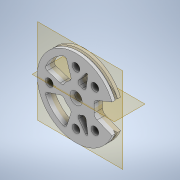
# Autodesk Inventor part: tendon_wh_2
Saved by Autodesk Inventor 2020 (Build 240168000, 168)
## iProperties
Created: 2020-12-06
Part Number: tendon_wh_2
Material: Generic
Document SubType Name: Modeling
Designer: Shuang Peng
Density: 1 g/cm^3
Appearance: Default
Mass: 3.1357 g
Surface Area: 22.5566 cm^2
Volume: 3.1357 cm^3
Author: Shuang Peng
Autodesk Inventor part; units mm, degrees
ref_plane "YZ Plane" through (0, 0, 0) normal (1, 0, 0) x (0, 1, 0)
ref_plane "XZ Plane" through (0, 0, 0) normal (0, 1, 0) x (-1, 0, 0)
ref_plane "XY Plane" through (0, 0, 0) normal (0, 0, 1) x (1, 0, 0)
sketch "Sketch1" plane through (0, 0, 0) normal (0, 0, 1) x (1, 0, 0)
  circle A0 centre (13.788582, -13.788582) radius 1.5
  circle A1 centre (0, 0) radius 3
  circle A2 centre (13.788582, -13.788582) radius 16
  point P0 (0, 0)
  dimension "d0" = 32
  constraints: 1 centre point, 1 coincident
  measures "d0" diameter of A2
extrude "Extrusion1" add sketch "Sketch1" along normal blind 3.5 contours A0 | A2
sketch "Sketch2" plane through (13.788582, -13.788582, 0) normal (0, 0, -1) x (-1, 0, 0)
  circle A0 centre (0, 0) radius 3.075
  line L0 (11.788582, 25.288582) -> (11.788582, 22.395184)
  line L1 (11.788582, 22.395184) -> (5.181981, 15.788582)
  line L2 (5.181981, 15.788582) -> (2.288582, 15.788582)
  arc A1 (2.288582, 15.788582) -> (0.510961, 14.705131) centre (2.288582, 13.788582) ccw
  line L3 (0.510961, 14.705131) -> (-7.071068, 0)
  line L4 (-7.071068, 0) -> (0, -7.071068)
  line L5 (0, -7.071068) -> (14.705131, 0.510961)
  arc A2 (14.705131, 0.510961) -> (15.788582, 2.288582) centre (13.788582, 2.288582) ccw
  line L6 (15.788582, 2.288582) -> (15.788582, 5.181981)
  line L7 (15.788582, 5.181981) -> (22.395184, 11.788582)
  line L8 (22.395184, 11.788582) -> (25.288582, 11.788582)
  arc A3 (25.288582, 11.788582) -> (25.288582, 15.788582) centre (25.288582, 13.788582) ccw
  line L9 (25.288582, 15.788582) -> (22.395184, 15.788582)
  line L10 (22.395184, 15.788582) -> (15.788582, 22.395184)
  line L11 (15.788582, 22.395184) -> (15.788582, 25.288582)
  arc A4 (15.788582, 25.288582) -> (11.788582, 25.288582) centre (13.788582, 25.288582) ccw
  circle A5 centre (13.788582, 25.288582) radius 1
  circle A6 centre (25.288582, 13.788582) radius 1
  circle A7 centre (13.788582, 13.788582) radius 5.15
  circle A8 centre (13.788582, 2.288582) radius 1
  circle A9 centre (2.288582, 13.788582) radius 1
  circle A10 centre (13.788582, 13.788582) radius 13.55
  circle A11 centre (0, 0) radius 4
  point P0 (13.788582, 13.788582)
  dimension "d3" = 8
  constraints: 1 centre point, 1 coincident
  measures "d3" diameter of A11
ref_plane "Work Plane1" through (5.684582, -20.85965, -8) normal (0, 0, 1) x (1, 0, 0)
extrude "Extrusion2" add sketch "Sketch2" along normal up to surface (8 mm away) contours A0 | A11
sketch "Sketch3" plane through (13.788582, -13.788582, -8) normal (0, 0, -1) x (-1, 0, 0)
  circle A0 centre (0, 0) radius 4 projected
  circle A1 centre (0, 0) radius 1.5
  point P0 (13.788582, 13.788582)
  dimension "d6" = 3
  constraints: 1 centre point, 1 coincident
  measures "d6" diameter of A1
extrude "Extrusion3" cut sketch "Sketch3" against normal blind 20 contours A1
ref_plane "Work Plane2" through (13.788582, -13.788582, 1.75) normal (0, 0, 1) x (1, 0, 0)
sketch "Sketch4" plane through (13.788582, -13.788582, 0) normal (0, 0, -1) x (-1, 0, 0)
  circle A0 centre (0, 0) radius 4 projected
  circle A1 centre (0, 0) radius 16 projected
  line L0 (0, 0) -> (10, 0)
  line L1 (11.5, 1.5) -> (8.5, 1.5)
  line L2 (8.5, 1.5) -> (8.5, -1.5)
  line L3 (8.5, -1.5) -> (11.5, -1.5)
  line L4 (11.5, -1.5) -> (11.5, 1.5)
  line L5 (11.5, 1.5) -> (8.5, -1.5) construction
  line L6 (8.5, 1.5) -> (11.5, -1.5) construction
  point P0 (13.788582, 13.788582)
  dimension "d9" = 10
  dimension "d10" = 3
  dimension "d11" = 3
  constraints: 14 end point, 2 midpoint, 2 parallel, 2 perpendicular, 1 horizontal
  measures "d9" distance of L0.start L0.end
  measures "d10" distance of L1.start L1.end
  measures "d11" distance of L2.end L1.end
extrude "Extrusion4" cut sketch "Sketch4" against normal blind 20 contours L4 L3 L2 L1
ref_plane "Work Plane3" through (2.288582, -13.788582, 0) normal (0, -1, 0) x (1, 0, 0)
sketch "Sketch5" plane through (2.288582, -13.788582, 0) normal (0, -1, 0) x (1, 0, 0)
  line L0 (27.5, 3.5) -> (-4.5, 3.5) projected
  line L1 (27.5, 0) -> (-4.5, 0) projected
  line L2 (-4.5, 0) -> (-4.5, 3.5)
  line L3 (-4.5, 0) -> (-4.5, 3.5) projected
  line L4 (-4.5, 1.75) -> (-4.5, 2.25)
  line L5 (-4.5, 1.75) -> (-4, 1.75)
  line L6 (-4.5, 1.75) -> (-4.5, 1.25)
  line L7 (-4.5, 1.25) -> (-4, 1.75)
  line L8 (-4.5, 2.25) -> (-4, 1.75)
  line L9 (15.5, 0) -> (7.5, 0) projected
  line L10 (7.5, -8) -> (15.5, -8) projected
  line L11 (11.5, 0) -> (11.5, -20)
  point P0 (-2.288582, 0)
  dimension "d15" = 0.5
  dimension "d16" = 0.5
  dimension "d17" = 0.5
  dimension "d18" = 20
  constraints: 14 end point, 2 midpoint, 2 point on line, 1 collinear, 1 horizontal, 1 vertical
  measures "d15" distance of L4.start L4.end
  measures "d16" distance of L4.start L5.end
  measures "d17" distance of L4.start L6.end
  measures "d18" distance of L11.start L11.end
revolve "Revolution1" cut sketch "Sketch5" angle 360 about axis through (13.788582, -13.788582, 0) along (0, 0, -1)
sketch "Sketch6" plane through (13.788582, -13.788582, 3.5) normal (0, 0, 1) x (1, 0, 0)
  line L0 (-11.5, 1.5) -> (-8.5, 1.5)
  line L1 (-8.5, 1.5) -> (-8.5, -1.5)
  line L2 (-8.5, -1.5) -> (-11.5, -1.5)
  line L3 (-11.5, -1.5) -> (-11.5, 1.5)
  circle A0 centre (0, 0) radius 1.5
  circle A1 centre (0, 0) radius 16
  line L4 (0, 0) -> (16, 0)
  line L5 (0, 0) -> (11.313708, -11.313708)
  line L6 (0, 0) -> (11.313708, 11.313708)
  line L7 (0, 0) -> (7.778175, -7.778175)
  circle A2 centre (7.778175, -7.778175) radius 1.6
  line L8 (0, 0) -> (7.778175, 7.778175)
  circle A3 centre (7.778175, 7.778175) radius 1.6
  point P0 (-13.788582, 13.788582)
  dimension "d20" = 45
  dimension "d21" = 45
  dimension "d22" = 11
  dimension "d23" = 3.2
  dimension "d24" = 11
  dimension "d25" = 3.2
  constraints: 10 end point, 3 point on circle, 2 centre point, 2 coincident, 2 point on line, 1 horizontal
  measures "d20" angle of L4 L5
  measures "d21" angle of L4 L6
  measures "d22" distance of L4.start L7.end
  measures "d23" diameter of A2
  measures "d24" distance of L4.start L8.end
  measures "d25" diameter of A3
extrude "Extrusion5" cut sketch "Sketch6" against normal blind 20 contours A3 L6 | L6 A3 | A2 L5 | L5 A2
sketch "Sketch7" plane through (13.788582, -13.788582, 3.5) normal (0, 0, 1) x (1, 0, 0)
  circle A0 centre (7.778175, 7.778175) radius 1.6
  circle A1 centre (7.778175, -7.778175) radius 1.6
  line L0 (-11.5, 1.5) -> (-8.5, 1.5)
  line L1 (-8.5, 1.5) -> (-8.5, -1.5)
  line L2 (-8.5, -1.5) -> (-11.5, -1.5)
  line L3 (-11.5, -1.5) -> (-11.5, 1.5)
  circle A2 centre (0, 0) radius 1.5
  circle A3 centre (0, 0) radius 16
  line L4 (0, 0) -> (16, 0)
  line L5 (0, 0) -> (14.834942, 5.993705)
  line L6 (0, 0) -> (14.834942, -5.993705)
  line L7 (7.417471, -2.996853) -> (7.417471, 2.996853)
  point P0 (-13.788582, 13.788582)
  dimension "d28" = 22
  dimension "d29" = 22
  constraints: 8 end point, 3 point on circle, 2 midpoint, 1 horizontal
  measures "d28" angle of L4 L6
  measures "d29" angle of L4 L5
extrude "Extrusion6" cut sketch "Sketch7" against normal blind 20 contours L7 L5 A3 L4 | L4 A3 L6 L7
fillet "Fillet1" radius 2 2 edges at (21.2061, -16.7854, 1.75) (21.2061, -10.7917, 1.75)
sketch "Sketch8" plane through (28.623524, -19.782288, 3.5) normal (0.3746066, 0.9271839, 0) x (0.9271839, -0.3746066, 0)
  line L0 (-6.650983, 0) -> (-6.650983, 3.5)
  line L1 (0, 0) -> (-6.650983, 0)
  line L2 (0, 1.25) -> (0, 0)
  line L3 (-0.5, 1.75) -> (0, 1.25)
  line L4 (0, 2.25) -> (-0.5, 1.75)
  line L5 (0, 3.5) -> (0, 2.25)
  line L6 (-6.650983, 3.5) -> (0, 3.5)
  line L7 (-0.5, 1.75) -> (-1.2, 1.75)
  line L8 (-31.5, 1.75) -> (-0.5, 1.75)
  line L9 (-1.2, 1.75) -> (0, 1.25)
  line L10 (0, 2.25) -> (-32, 2.25)
  line L11 (-1.2, 1.75) -> (0, 2.25)
  point P0 (-33.949845, 3.5)
  point P1 (-4.850233, 1.75)
  point P2 (-4.490563, 2.25)
  dimension "d33" = 0.7
  constraints: 6 end point, 1 point on line
  measures "d33" distance of L3.start L7.end
extrude "Extrusion7" cut sketch "Sketch8" against normal blind 20 contours L11 L4 L7 | L7 L3 L9
sketch "Sketch9" plane through (28.623524, -7.794877, 0) normal (0.3746066, -0.9271839, 0) x (0.9271839, 0.3746066, 0)
  line L0 (-6.650983, 0) -> (-6.650983, 3.5)
  line L1 (0, 0) -> (-6.650983, 0)
  line L2 (0, 1.25) -> (0, 0)
  line L3 (-0.5, 1.75) -> (0, 1.25)
  line L4 (0, 2.25) -> (-0.5, 1.75)
  line L5 (0, 3.5) -> (0, 2.25)
  line L6 (-6.650983, 3.5) -> (0, 3.5)
  line L7 (-0.5, 1.75) -> (-1.2, 1.75)
  line L8 (-0.5, 1.75) -> (-31.5, 1.75)
  line L9 (-1.2, 1.75) -> (0, 2.25)
  line L10 (-32, 1.25) -> (0, 1.25)
  line L11 (-1.2, 1.75) -> (0, 1.25)
  point P0 (-23.619257, 0)
  point P1 (-8.552973, 1.75)
  point P2 (-4.490563, 1.25)
  dimension "d36" = 0.7
  constraints: 6 end point, 1 point on line
  measures "d36" distance of L3.start L7.end
extrude "Extrusion8" cut sketch "Sketch9" against normal blind 20 contours L11 L7 L3 | L9 L4 L7
sketch "Sketch10" plane through (0, 0, 0) normal (0, 0, -1) x (-1, 0, 0)
  arc A0 (-25.785678, -23.602842) -> (-25.785678, -3.974323) centre (-13.788582, -13.788582) ccw
  line L0 (-13.788582, -13.788582) -> (-13.788582, -2.788582)
  circle A1 centre (-13.788582, -2.788582) radius 1.6
  line L1 (-13.788582, -13.788582) -> (-13.788582, -24.788582)
  circle A2 centre (-13.788582, -24.788582) radius 1.6
  point P0 (0, 0)
  dimension "d41" = 11
  dimension "d42" = 3.2
  dimension "d43" = 11
  dimension "d44" = 3.2
  constraints: 4 end point, 2 centre point, 2 coincident, 2 vertical
  measures "d41" distance of L0.start L0.end
  measures "d42" diameter of A1
  measures "d43" distance of L0.start L1.end
  measures "d44" diameter of A2
extrude "Extrusion9" cut sketch "Sketch10" against normal blind 20
sketch "Sketch11" plane through (0, 0, 3.5) normal (0, 0, 1) x (1, 0, 0)
  circle A0 centre (13.788582, -2.788582) radius 1.6
  circle A1 centre (13.788582, -24.788582) radius 1.6
  line L0 (28.623524, -19.782288) -> (22.45684, -17.290786)
  arc A2 (21.206053, -15.436418) -> (22.45684, -17.290786) centre (23.206053, -15.436418) ccw
  line L1 (21.206053, -15.436418) -> (21.206053, -12.140747)
  arc A3 (22.45684, -10.286379) -> (21.206053, -12.140747) centre (23.206053, -12.140747) ccw
  line L2 (22.45684, -10.286379) -> (28.623524, -7.794877)
  arc A4 (28.623524, -7.794877) -> (28.623524, -19.782288) centre (13.788582, -13.788582) ccw
  circle A5 centre (13.788582, -13.788582) radius 1.5
  line L3 (2.288582, -12.288582) -> (5.288582, -12.288582)
  line L4 (5.288582, -12.288582) -> (5.288582, -15.288582)
  line L5 (5.288582, -15.288582) -> (2.288582, -15.288582)
  line L6 (2.288582, -15.288582) -> (2.288582, -12.288582)
  circle A6 centre (21.566757, -21.566757) radius 1.6
  circle A7 centre (21.566757, -6.010408) radius 1.6
  point P0 (0, 0)
extrude "Extrusion10" add sketch "Sketch11" against normal up to surface (3.5 mm away) contours L3 L4 L5 L6
sketch "Sketch12" plane through (0, 0, 0) normal (0, 0, -1) x (-1, 0, 0)
  circle A0 centre (-13.788582, -2.788582) radius 1.6
  circle A1 centre (-13.788582, -24.788582) radius 1.6
  line L0 (-22.45684, -17.290786) -> (-28.623524, -19.782288)
  arc A2 (-28.623524, -19.782288) -> (-28.623524, -7.794877) centre (-13.788582, -13.788582) ccw
  line L1 (-28.623524, -7.794877) -> (-22.45684, -10.286379)
  arc A3 (-21.206053, -12.140747) -> (-22.45684, -10.286379) centre (-23.206053, -12.140747) ccw
  line L2 (-21.206053, -12.140747) -> (-21.206053, -15.436418)
  arc A4 (-22.45684, -17.290786) -> (-21.206053, -15.436418) centre (-23.206053, -15.436418) ccw
  circle A5 centre (-21.566757, -6.010408) radius 1.6
  circle A6 centre (-21.566757, -21.566757) radius 1.6
  circle A7 centre (-13.788582, -13.788582) radius 4
  line L3 (-13.788582, -13.788582) -> (-2.788582, -13.788582)
  circle A8 centre (-2.788582, -13.788582) radius 1.6
  point P0 (0, 0)
  dimension "d49" = 11
  dimension "d50" = 3.2
  constraints: 2 end point, 1 centre point, 1 coincident, 1 horizontal
  measures "d49" distance of L3.start L3.end
  measures "d50" diameter of A8
extrude "Extrusion11" cut sketch "Sketch12" against normal blind 20 contours A8
sketch "Sketch13" plane through (0, 0, 0) normal (0, 0, -1) x (-1, 0, 0)
  circle A0 centre (-2.788582, -13.788582) radius 1.6
  circle A1 centre (-13.788582, -2.788582) radius 1.6
  circle A2 centre (-13.788582, -24.788582) radius 1.6
  line L0 (-22.45684, -17.290786) -> (-28.623524, -19.782288)
  arc A3 (-28.623524, -19.782288) -> (-28.623524, -7.794877) centre (-13.788582, -13.788582) ccw
  line L1 (-28.623524, -7.794877) -> (-22.45684, -10.286379)
  arc A4 (-21.206053, -12.140747) -> (-22.45684, -10.286379) centre (-23.206053, -12.140747) ccw
  line L2 (-21.206053, -12.140747) -> (-21.206053, -15.436418)
  arc A5 (-22.45684, -17.290786) -> (-21.206053, -15.436418) centre (-23.206053, -15.436418) ccw
  circle A6 centre (-21.566757, -6.010408) radius 1.6
  circle A7 centre (-21.566757, -21.566757) radius 1.6
  circle A8 centre (-13.788582, -13.788582) radius 4
  arc A9 (-25.785678, -23.602842) -> (-25.785678, -3.974323) centre (-13.788582, -13.788582) ccw
  circle A10 centre (-13.788582, -13.788582) radius 13.5
  circle A11 centre (-13.788582, -13.788582) radius 5.5
  line L3 (-13.788582, -13.788582) -> (-13.788582, -2.788582)
  line L4 (-13.788582, -13.788582) -> (-2.788582, -13.788582)
  line L5 (-13.788582, -13.788582) -> (-9.616853, -0.949319)
  line L6 (-13.788582, -13.788582) -> (-13.788582, -24.788582)
  line L7 (-13.788582, -13.788582) -> (-0.949319, -9.616853)
  line L8 (-13.788582, -13.788582) -> (-0.949319, -17.960312)
  line L9 (-13.788582, -13.788582) -> (-9.616853, -26.627845)
  point P0 (0, 0)
  point P1 (-12.088989, -19.019393)
  point P2 (-8.557771, -15.488176)
  point P3 (-8.557771, -12.088989)
  point P4 (-12.088989, -8.557771)
  dimension "d53" = 27
  dimension "d54" = 11
  dimension "d55" = 18
  dimension "d56" = 18
  dimension "d57" = 18
  dimension "d58" = 18
  constraints: 14 end point, 4 point on circle, 2 centre point, 2 coincident, 2 vertical, 1 horizontal
  measures "d53" diameter of A10
  measures "d54" diameter of A11
  measures "d55" angle of L3 L5
  measures "d56" angle of L4 L7
  measures "d57" angle of L4 L8
  measures "d58" angle of L6 L9
extrude "Extrusion12" cut sketch "Sketch13" against normal blind 20 contours L9 A11 L8 A10 | A10 L7 A11 L5
fillet "Fillet2" radius 1.5 4 edges at (8.5578, -12.089, 1.75) (12.089, -19.0194, 1.75) (8.5578, -15.4882, 1.75) (12.089, -8.5578, 1.75)
fillet "Fillet2" radius 1 4 edges at (9.6169, -26.6278, 1.75) (0.9493, -17.9603, 1.75) (0.9493, -9.6169, 1.75) (9.6169, -0.9493, 1.75)
chamfer "Chamfer1" distance 1 angle 45 1 edges at (15.2886, -13.7886, 3.5)
sketch "Sketch14" plane through (0, 0, 3.5) normal (0, 0, 1) x (1, 0, 0)
  circle A0 centre (21.566757, -6.010408) radius 1.6
  circle A1 centre (21.566757, -21.566757) radius 1.6
  line L0 (28.623524, -19.782288) -> (22.45684, -17.290786)
  arc A2 (21.206053, -15.436418) -> (22.45684, -17.290786) centre (23.206053, -15.436418) ccw
  line L1 (21.206053, -15.436418) -> (21.206053, -12.140747)
  arc A3 (22.45684, -10.286379) -> (21.206053, -12.140747) centre (23.206053, -12.140747) ccw
  line L2 (22.45684, -10.286379) -> (28.623524, -7.794877)
  arc A4 (28.623524, -7.794877) -> (28.623524, -19.782288) centre (13.788582, -13.788582) ccw
  circle A5 centre (13.788582, -24.788582) radius 1.6
  circle A6 centre (13.788582, -2.788582) radius 1.6
  circle A7 centre (2.788582, -13.788582) radius 1.6
  line L3 (9.93825, -1.938479) -> (11.67571, -7.285831)
  arc A8 (11.007581, -9.043476) -> (11.67571, -7.285831) centre (10.249126, -7.749357) ccw
  arc A9 (11.007581, -9.043476) -> (9.043476, -11.007581) centre (13.788582, -13.788582) ccw
  arc A10 (7.285831, -11.67571) -> (9.043476, -11.007581) centre (7.749357, -10.249126) ccw
  line L4 (7.285831, -11.67571) -> (1.938479, -9.93825)
  arc A11 (1.324209, -8.603083) -> (1.938479, -9.93825) centre (2.247496, -8.987194) ccw
  arc A12 (8.603083, -1.324209) -> (1.324209, -8.603083) centre (13.788582, -13.788582) ccw
  arc A13 (9.93825, -1.938479) -> (8.603083, -1.324209) centre (8.987194, -2.247496) ccw
  arc A14 (1.324209, -18.974082) -> (8.603083, -26.252955) centre (13.788582, -13.788582) ccw
  arc A15 (1.938479, -17.638914) -> (1.324209, -18.974082) centre (2.247496, -18.589971) ccw
  line L5 (1.938479, -17.638914) -> (7.285831, -15.901454)
  arc A16 (9.043476, -16.569584) -> (7.285831, -15.901454) centre (7.749357, -17.328039) ccw
  arc A17 (9.043476, -16.569584) -> (11.007581, -18.533688) centre (13.788582, -13.788582) ccw
  arc A18 (11.67571, -20.291333) -> (11.007581, -18.533688) centre (10.249126, -19.827808) ccw
  line L6 (11.67571, -20.291333) -> (9.93825, -25.638685)
  arc A19 (8.603083, -26.252955) -> (9.93825, -25.638685) centre (8.987194, -25.329668) ccw
  circle A20 centre (13.788582, -13.788582) radius 2.5
  circle A21 centre (13.788582, -13.788582) radius 5.5
  line L7 (21.566757, -21.566757) -> (13.788582, -24.788582)
  circle A22 centre (13.788582, -13.788582) radius 2.5
  line L8 (13.788582, -13.788582) -> (17.67767, -23.17767)
  line L9 (13.788582, -13.788582) -> (18.954809, -26.260956)
  line L10 (13.788582, -13.788582) -> (13.788582, -24.788582)
  line L11 (13.788582, -13.788582) -> (21.566757, -21.566757)
  line L12 (18.954809, -26.260956) -> (13.788582, -19.288582)
  line L13 (18.954809, -26.260956) -> (17.67767, -17.67767)
  point P0 (0, 0)
  point P1 (13.788582, -19.288582)
  point P2 (17.67767, -17.67767)
  dimension "d66" = 11
  dimension "d67" = 13.5
  constraints: 14 end point, 3 midpoint, 1 centre point, 1 coincident, 1 perpendicular, 1 vertical
  measures "d66" diameter of A21
  measures "d67" distance of L8.start L9.end
extrude "Extrusion13" cut sketch "Sketch14" against normal blind 20 contours L13 L7 L8 A21 | L13 L9 L7 | L8 L7 L12 A21 | L9 L12 L7
fillet "Fillet3" radius 0.5 1 edges at (18.9548, -26.261, 1.75)
fillet "Fillet4" radius 1 2 edges at (13.7886, -19.2886, 1.75) (17.6777, -17.6777, 1.75)
ref_plane "Work Plane4" through (13.788582, -13.788582, 3.5) normal (0, 1, 0) x (0, 0, 1)
mirror "Mirror1" about plane through (13.788582, -13.788582, 3.5) normal (0, 1, 0) of "Extrusion13", "Fillet3", "Fillet4"
fillet "Fillet5" radius 1.5 1 edges at (17.7886, -13.7886, 0)
body "Solid1"
